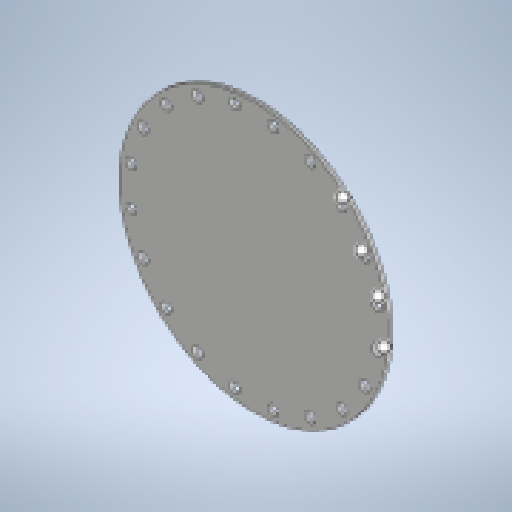
# Autodesk Inventor part: PRS 1621 charging hatch D1200
Saved by Autodesk Inventor 2026.2 (Build 302298000, 298)
## iProperties
Created: 2025-02-12
Part Number: PRS 1621 charging hatch D1200
Material: Generic
Document SubType Name: Sheet Metal
Designer: admin
Density: 1 g/cm^3
Flat Pattern Width: 67 cm
Flat Pattern Length: 67 cm
Flat Pattern Area: 4489 cm^2
Sheet Metal Rule: Default_mm
Sheet Metal Width: 670,000 mm
Sheet Metal Length: 670,000 mm
Sheet Metal Area: 448900,000 mm^2
Appearance: Default
Author: pokla
Autodesk Inventor part; units mm, degrees
ref_plane "YZ Plane" through (0, 0, 0) normal (1, 0, 0) x (0, 1, 0)
ref_plane "XZ Plane" through (0, 0, 0) normal (0, 1, 0) x (-1, 0, 0)
ref_plane "XY Plane" through (0, 0, 0) normal (0, 0, 1) x (1, 0, 0)
sketch "Sketch1" plane through (0, 0, 0) normal (0, 1, 0) x (-1, 0, 0)
  circle A0 centre (0, 0) radius 335
  dimension "d0" = 670
  constraints: 1 centre point, 1 coincident
  measures "d0" diameter of A0
extrude "Extrusion1" add sketch "Sketch1" along normal blind 10
sketch "Sketch2" plane through (0, 10, 0) normal (0, 1, 0) x (1, 0, 0)
  circle A0 centre (0, 0) radius 310 construction
  line L0 (0, 0) -> (-310, 0)
  line L1 (0, 0) -> (-306.1834, 48.4947) construction
  point P0 (-306.1834, -48.4947)
  point P1 (-306.1834, -48.4947)
  point P2 (-276.212, -140.7371)
  point P3 (-276.212, -140.7371)
  point P4 (-219.2031, -219.2031)
  point P5 (-219.2031, -219.2031)
  point P6 (-140.7371, -276.212)
  point P7 (-140.7371, -276.212)
  point P8 (-48.4947, -306.1834)
  point P9 (-48.4947, -306.1834)
  point P10 (48.4947, -306.1834)
  point P11 (48.4947, -306.1834)
  point P12 (140.7371, -276.212)
  point P13 (140.7371, -276.212)
  point P14 (219.2031, -219.2031)
  point P15 (219.2031, -219.2031)
  point P16 (276.212, -140.7371)
  point P17 (276.212, -140.7371)
  point P18 (306.1834, -48.4947)
  point P19 (306.1834, -48.4947)
  point P20 (306.1834, 48.4947)
  point P21 (306.1834, 48.4947)
  point P22 (276.212, 140.7371)
  point P23 (276.212, 140.7371)
  point P24 (219.2031, 219.2031)
  point P25 (219.2031, 219.2031)
  point P26 (140.7371, 276.212)
  point P27 (140.7371, 276.212)
  point P28 (48.4947, 306.1834)
  point P29 (48.4947, 306.1834)
  point P30 (-48.4947, 306.1834)
  point P31 (-48.4947, 306.1834)
  point P32 (-140.7371, 276.212)
  point P33 (-140.7371, 276.212)
  point P34 (-219.2031, 219.2031)
  point P35 (-219.2031, 219.2031)
  point P36 (-276.212, 140.7371)
  point P37 (-276.212, 140.7371)
  dimension "d4" = 620
  dimension "d11" = 9
  dimension "d24" = 360
  constraints: 21 coincident, 4 end point, 2 point on circle, 1 centre point, 1 horizontal, 41 other
  measures "d4" diameter of A0
  measures "d11" angle of L0 L1
hole "Hole2" at (-306.1834, 10, -48.4947) at (-306.1834, 10, 48.4947) at (-276.212, 10, 140.7371) at (-219.2031, 10, 219.2031) at (-140.7371, 10, 276.212) at (-48.4947, 10, 306.1834) at (48.4947, 10, 306.1834) at (140.7371, 10, 276.212) at (219.2031, 10, 219.2031) at (276.212, 10, 140.7371) at (306.1834, 10, 48.4947) at (306.1834, 10, -48.4947) at (276.212, 10, -140.7371) at (219.2031, 10, -219.2031) at (140.7371, 10, -276.212) at (48.4947, 10, -306.1834) at (-48.4947, 10, -306.1834) at (-140.7371, 10, -276.212) at (-219.2031, 10, -219.2031) at (-276.212, 10, -140.7371) direction (0, -1, 0) diameter 26 end through all
equation "\"d1\" = Thickness"
equation "\"BendReliefDepth\" = 0.5 * Thickness"
equation "\"Thickness\" = 10"
body "Solid1"
